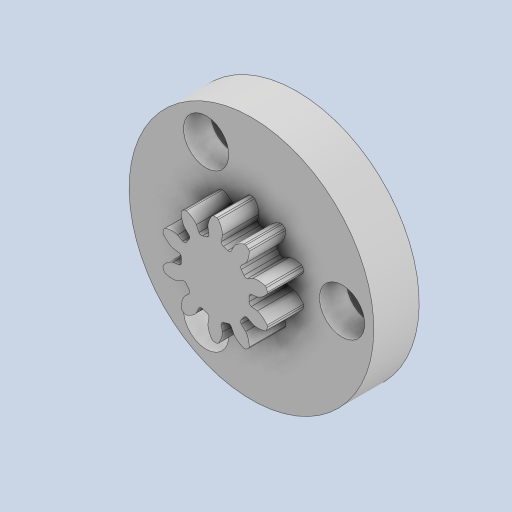
# Autodesk Inventor part: tyuusinn
Saved by Autodesk Inventor 2023 (Build 270158000, 158)
## iProperties
Created: 2024-11-27
Part Number: tyuusinn
Material: Generic
Document SubType Name: Modeling
Designer: kiyo
Density: 1 g/cm^3
Appearance: Default
Author: kiyo
Autodesk Inventor part; units mm, degrees
ref_plane "YZ Plane" through (0, 0, 0) normal (1, 0, 0) x (0, 1, 0)
ref_plane "XZ Plane" through (0, 0, 0) normal (0, 1, 0) x (-1, 0, 0)
ref_plane "XY Plane" through (0, 0, 0) normal (0, 0, 1) x (1, 0, 0)
sketch "スケッチ3" plane through (0, 0, 0) normal (1, 0, 0) x (0, 1, 0)
  circle A0 centre (0, 0) radius 5
  circle A1 centre (0, 0) radius 4.6985
  line L0 (0, 0) -> (4.6511, 0.6658)
  line L1 (0, 0) -> (4.9384, 0.7822)
  line L2 (0, 0) -> (7.1132, 0)
  dimension "d12" = 10
  dimension "d13" = 9.3969
  dimension "d17" = 9
  constraints: 6 end point, 2 coincident, 1 horizontal, 11 other
  measures "d17" angle of L2 L1
sketch "スケッチ4" plane through (0, 0, 0) normal (1, 0, 0) x (0, 1, 0)
  circle A0 centre (0, 0) radius 6
  dimension "d18" = 12
  constraints: 1 centre point, 1 coincident
  measures "d18" diameter of A0
extrude "押し出し3" add sketch "スケッチ4" along normal blind 4
sketch "スケッチ5" plane through (4, 0, 0) normal (1, 0, 0) x (0, 0, -1)
  circle A0 centre (0, 0) radius 6 projected
  line L0 (0, 0) -> (-0.6658, 4.6511) projected
  spline S0 degree 3 poles (-0.6658, 4.6511) (-0.6658, 4.6511) (-0.7403, 5.0598) (-1.2941, 5.5629) (-1.5415, 5.7877) (-1.8807, 6.0252) (-2.3207, 6.2262) knots 0 0 0 0 0.691133 0.691133 0.691133 1 1 1 1 projected
  circle A1 centre (0, 0) radius 3.75
  line L1 (0, 0) -> (0, 6)
  point P0 (0, 3.75)
  point P1 (-1.5726, 5.7902)
  point P2 (-0.5314, 3.7122)
  dimension "d21" = 7.5
  constraints: 2 end point, 1 centre point, 1 coincident, 1 vertical, 2 other
  measures "d21" diameter of A1
extrude "押し出し4" cut sketch "スケッチ5" against normal blind 4 contours L1 A1 L0 S0 A0 picked at (-0.2219, 4.8004)
fillet "フィレット1" radius 0.3 1 edges at (2, 3.7122, 0.5314)
chamfer "面取り1" distance 0.1 angle 45 1 edges at (2, 5.7902, 1.5726)
mirror "ミラー1" about plane through (4, 6, 0) normal (0, 0, 1) of "押し出し4", "フィレット1", "面取り1"
pattern_circular "円形状パターン1" count 10 over 360 about axis through (0, 0, 0) along (1, 0, 0) of "押し出し4", "フィレット1", "面取り1", "ミラー1"
sketch "スケッチ6" plane through (0, 0, 0) normal (-1, 0, 0) x (0, 0, 1)
  circle A0 centre (0, 0) radius 13.5
  circle A1 centre (0, 10) radius 1.35
  line L0 (0, 0) -> (0, 12.5713)
  circle A2 centre (-8.6603, -5) radius 1.35
  circle A3 centre (8.6603, -5) radius 1.35
  dimension "d31" = 27
  dimension "d32" = 2.7
  dimension "d33" = 10
  dimension "d36" = 360
  constraints: 4 centre point, 2 end point, 1 coincident, 1 point on line, 1 vertical, 7 other
  measures "d31" diameter of A0
  measures "d32" diameter of A1
  measures "d33" distance of point (0, 0) A1.centre
extrude "押し出し5" add sketch "スケッチ6" along normal blind 5
sketch "スケッチ7" plane through (0, 0, 0) normal (1, 0, 0) x (0, 0, -1)
  circle A0 centre (8.6603, -5) radius 1.35 projected
  circle A1 centre (8.6603, -5) radius 2.5
  circle A2 centre (0, 0) radius 13.5 projected
  circle A3 centre (0, 10) radius 2.5
  circle A4 centre (-8.6603, -5) radius 2.5
  dimension "d40" = 5
  dimension "d43" = 360
  constraints: 3 centre point, 1 coincident, 7 other
  measures "d40" diameter of A1
extrude "押し出し6" cut sketch "スケッチ7" against normal blind 3 contours A1 | A3 | A4
equation "\"module\" = 1"
